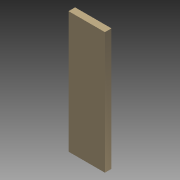
# Autodesk Inventor part: Z plate
Saved by Autodesk Inventor 2012 (Build 160160000, 160)
## iProperties
Created: 2013-05-09
Part Number: Z plate
Material: Default
Document SubType Name: Modeling
Designer: Fabian
Density: 1 g/cm^3
Author: Fabian
Autodesk Inventor part; units mm, degrees
ref_plane "YZ Plane" through (0, 0, 0) normal (1, 0, 0) x (0, 1, 0)
ref_plane "XZ Plane" through (0, 0, 0) normal (0, 1, 0) x (-1, 0, 0)
ref_plane "XY Plane" through (0, 0, 0) normal (0, 0, 1) x (1, 0, 0)
sketch "Sketch1" plane through (0, 0, 0) normal (0, 0, 1) x (1, 0, 0)
  line L0 (-21.049, 4.8951) -> (84.361, 4.8951)
  line L1 (84.361, 4.8951) -> (84.361, -347.5049)
  line L2 (84.361, -347.5049) -> (-21.049, -347.5049)
  line L3 (-21.049, -347.5049) -> (-21.049, 4.8951)
  point P0 (0, 0)
  dimension "d0" = 105.41
  dimension "d1" = 352.4
  constraints: 8 end point, 2 parallel, 1 horizontal, 1 perpendicular
  measures "d0" distance of L0.start L0.end
  measures "d1" distance of L2.end L0.start
extrude "Extrusion1" add sketch "Sketch1" along normal blind 19.05
body "Solid1"
